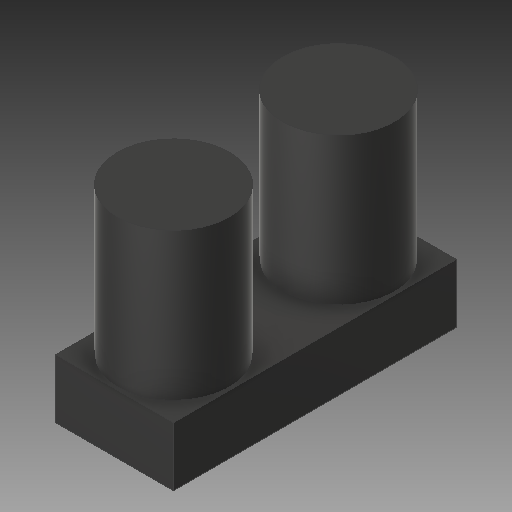
# Autodesk Inventor part: LIDARLite
Saved by Autodesk Inventor 2018 (Build 220112000, 112)
## iProperties
Created: 2017-10-07
Part Number: LIDARLite
Material: Acetal Resin, Black
Document SubType Name: Modeling
Designer: Akram Al-Hourani
Density: 1.425 g/cm^3
Appearance: Smooth - Black
Author: Akram Al-Hourani
Autodesk Inventor part; units mm, degrees
ref_plane "YZ Plane" through (0, 0, 0) normal (1, 0, 0) x (0, 1, 0)
ref_plane "XZ Plane" through (0, 0, 0) normal (0, 1, 0) x (-1, 0, 0)
ref_plane "XY Plane" through (0, 0, 0) normal (0, 0, 1) x (1, 0, 0)
sketch "Sketch1" plane through (0, 0, 0) normal (0, 1, 0) x (-1, 0, 0)
  line L0 (-10, 24) -> (10, 24)
  line L1 (10, 24) -> (10, -24)
  line L2 (10, -24) -> (-10, -24)
  line L3 (-10, -24) -> (-10, 24)
  line L4 (-10, 24) -> (10, -24) construction
  line L5 (10, 24) -> (-10, -24) construction
  line L6 (0, 0) -> (0, -23.5) construction
  line L7 (0, -23.5) -> (0, -14) construction
  circle A0 centre (0, -14) radius 9.5
  line L8 (0, 0) -> (0, 23.5) construction
  line L9 (0, 23.5) -> (0, 14) construction
  circle A1 centre (0, 14) radius 9.5
  dimension "d0" = 20
  dimension "d1" = 48
  dimension "d2" = 23.5
  dimension "d3" = 9.5
  dimension "d4" = 19
  dimension "d5" = 23.5
  dimension "d6" = 9.5
  dimension "d7" = 19
  constraints: 20 end point, 3 point on line, 2 centre point, 2 coincident, 2 midpoint, 2 parallel, 1 horizontal, 1 perpendicular, 1 vertical
  measures "d0" distance of L1.end L2.end
  measures "d1" distance of L0.end L1.end
  measures "d2" distance of L6.start L6.end
  measures "d3" distance of L6.end L7.end
  measures "d4" diameter of A0
  measures "d5" distance of L6.start L8.end
  measures "d6" distance of L8.end L9.end
  measures "d7" diameter of A1
extrude "Extrusion1" add sketch "Sketch1" along normal blind 25 contours A0 | A1
extrude "Extrusion2" add sketch "Sketch1" against normal blind 10
extrude "Extrusion3" add sketch "Sketch1" against normal blind 10 contours A1
extrude "Extrusion4" add sketch "Sketch1" against normal blind 10 contours A0
body "Solid1"
